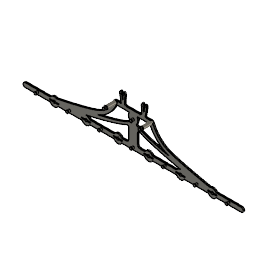
Piesa_4_cadru_sustinere (Autodesk Fusion 360 design; units mm, degrees)
part number: 2026-05-31-10-45-45-037
part number: 2026-05-31-14-30-49-266
Autodesk Fusion 360 part; units mm, degrees
sketch "top view" plane through (0, 0, 0) normal (0, 0, 1) x (1, 0, 0)
  line L0 (-248.6196, 9.3522) -> (-127.5156, 9.3522) construction
  line L1 (-248.6196, 9.3522) -> (-248.6196, 11.8522) construction
  arc A0 (-248.6196, 11.8522) -> (-249.2773, 6.9403) centre (-248.6196, 9.3522) ccw
  line L2 (-248.6196, 9.3522) -> (-216.3996, 9.3522) construction
  line L3 (-128.1733, 26.3643) -> (-128.1733, 29.0223) construction
  line L4 (-148.1733, 45.1233) -> (-148.1733, 43.1233) construction
  line L5 (-216.3996, 9.3522) -> (-216.3996, 13.6062) construction
  line L6 (-216.3996, 13.6062) -> (-213.7722, 13.6062) construction
  line L7 (-128.1733, 29.0223) -> (-180, 29.0223) construction
  spline S0 degree 5 poles (-213.7722, 13.6062) (-211.7009, 14.0329) (-207.6293, 14.8839) (-201.7349, 16.1535) (-194.3087, 17.832) (-185.8111, 19.9044) (-178.2122, 21.9474) (-171.6715, 23.9556) (-166.7674, 25.7797) (-163.881, 27.1788) (-162.3464, 28.1749) (-161.6154, 28.7858) (-161.3648, 29.0223) knots 0 0 0 0 0 0 0.1 0.2 0.3 0.4 0.5 0.6 0.7 0.76362 0.76362 0.76362 0.76362 0.76362 0.76362
  line L8 (-162.8508, 27.6198) -> (-159.8789, 30.4247)
  arc A1 (-170.1166, 24.5955) -> (-150.0471, 43.8225) centre (-180, 55) ccw
  line L9 (-132.8823, 41.1233) -> (-146.814, 41.1233)
  arc A2 (-148.1733, 45.1233) -> (-150.0471, 43.8225) centre (-148.1733, 43.1233) ccw
  line L10 (-128.1733, 41.1233) -> (-128.1733, 37.7953) construction
  line L11 (-128.1733, 35.7263) -> (-131.5853, 35.7263) construction
  line L12 (-128.1733, 41.1233) -> (-145.1293, 41.1233) construction
  line L13 (-145.1293, 41.1233) -> (-145.1293, 29.0223) construction
  line L14 (-180.8396, 9.3522) -> (-180.8396, 18.8752) construction
  line L15 (-180.8396, 18.8752) -> (-179.7346, 18.8752) construction
  arc A3 (-132.8823, 41.1233) -> (-131.5853, 32.7598) centre (-125.2153, 38.03) ccw
  arc A4 (-167.1807, 21.3913) -> (-165.0411, 22.2875) centre (-180, 55) ccw
  arc A5 (-158.8318, 25.9177) -> (-146.814, 41.1233) centre (-180, 55) ccw
  spline S1 degree 3 poles (-165.0411, 22.2875) (-163.9439, 22.76) (-162.9356, 23.2427) (-162.0149, 23.7457) (-160.8198, 24.3987) (-159.766, 25.0783) (-158.8318, 25.9177) knots 0.602738 0.602738 0.602738 0.602738 0.669843 0.669843 0.669843 0.756952 0.756952 0.756952 0.756952
  line L16 (-167.3845, 21.3116) -> (-167.4008, 21.3082)
  line L17 (-128.1733, 9.3522) -> (-128.1733, 26.3643) construction
  line L18 (-128.1733, 26.3643) -> (-134.6583, 26.3643) construction
  line L19 (-128.1733, 27.8213) -> (-135.0433, 27.8213) construction
  line L20 (-133.1518, 26.3643) -> (-133.1518, 2) construction
  arc A6 (-133.1518, 26.3643) -> (-135.0504, 27.8188) centre (-134.6583, 26.3643) ccw
  spline S2 degree 3 poles (-135.0504, 27.8188) (-135.0481, 27.8196) (-135.0457, 27.8204) (-135.0433, 27.8213) knots 0.499817 0.499817 0.499817 0.499817 0.499919 0.499919 0.499919 0.499919
  spline S3 degree 5 poles (-167.641, 21.24) (-166.401, 21.5014) (-163.424, 22.1424) (-158.8454, 23.181) (-152.9154, 24.6505) (-146.0504, 26.6065) (-140.0833, 28.6496) (-136.0679, 30.3417) (-133.5388, 31.6209) (-132.1186, 32.4368) (-131.5853, 32.7598) knots 0.130161 0.130161 0.130161 0.130161 0.130161 0.130161 0.2 0.3 0.4 0.5 0.6 0.664497 0.664497 0.664497 0.664497 0.664497 0.664497
  line L21 (-172.5766, 20.1992) -> (-162.7054, 22.2807)
  line L22 (-133.8581, 31.3829) -> (-129.3125, 34.1368)
  line L23 (-167.641, 21.24) -> (-167.1807, 21.3913)
  spline S4 degree 5 poles (-167.5607, 21.2747) (-167.5468, 21.2776) (-167.5328, 21.2805) (-167.5189, 21.2835) (-167.505, 21.2864) (-167.491, 21.2893) knots 0.123283 0.123283 0.123283 0.123283 0.123283 0.123283 0.124016 0.124016 0.124016 0.124016 0.124016 0.124016
  line L24 (-167.5678, 21.2732) -> (-167.5536, 21.2762)
  line L25 (-167.4981, 21.2878) -> (-167.4839, 21.2908)
  spline S5 degree 5 poles (-180.8396, 14.3522) (-179.0351, 14.7525) (-175.4777, 15.5549) (-170.2971, 16.764) (-163.7053, 18.3875) (-156.0341, 20.4372) (-149.0013, 22.5098) (-143.3292, 24.3981) (-139.4226, 25.8848) (-136.9109, 26.9566) (-135.5066, 27.6032) (-135.0504, 27.8188) knots 0 0 0 0 0 0 0.1 0.2 0.3 0.4 0.5 0.6 0.649903 0.649903 0.649903 0.649903 0.649903 0.649903
  line L26 (-138.104, 26.3752) -> (-131.9968, 29.2625)
  line L27 (-133.1518, 26.3643) -> (-133.1518, 14.3522)
  line L28 (-249.2773, 6.9403) -> (-220.7794, 6.9403)
  line L29 (-248.6196, 11.8522) -> (-220.7297, 11.8522)
  line L30 (-212.0198, 6.9403) -> (-185.2194, 6.9403)
  arc A7 (-185.2194, 6.9403) -> (-176.4598, 6.9403) centre (-180.8396, 9.3522) ccw
  arc A8 (-176.5095, 11.8522) -> (-180.8396, 14.3522) centre (-180.8396, 9.3522) ccw
  line L31 (-176.5095, 11.8522) -> (-149.6097, 11.8522)
  line L32 (-176.4598, 6.9403) -> (-149.6594, 6.9403)
  line L33 (-140.8998, 6.9403) -> (-128.1733, 6.9403)
  arc A9 (-149.6594, 6.9403) -> (-140.8998, 6.9403) centre (-145.2796, 9.3522) ccw
  arc A10 (-140.9495, 11.8522) -> (-149.6097, 11.8522) centre (-145.2796, 9.3522) ccw
  line L34 (-140.9495, 11.8522) -> (-135.6518, 11.8522)
  arc A11 (-135.6518, 11.8522) -> (-133.1518, 14.3522) centre (-135.6518, 14.3522) ccw
  arc A12 (-213.7722, 13.6062) -> (-220.7297, 11.8522) centre (-216.3996, 9.3522) ccw
  arc A13 (-220.7794, 6.9403) -> (-212.0198, 6.9403) centre (-216.3996, 9.3522) ccw
  line L35 (-128.1733, 45.1233) -> (-136.1553, 45.1233) construction
  line L36 (-148.1733, 45.1233) -> (-141.5903, 45.1233) construction
  line L37 (-136.1553, 45.1233) -> (-136.1553, 46.6233) construction
  line L38 (-140.4243, 45.1233) -> (-140.4243, 50.0803) construction
  line L39 (-140.4243, 50.0803) -> (-139.9633, 50.0803) construction
  line L40 (-140.4243, 50.0803) -> (-140.5759, 53.5518)
  line L41 (-140.4243, 50.0803) -> (-136.9203, 50.0803) construction
  line L42 (-139.5023, 50.0803) -> (-139.8213, 53.5851)
  line L43 (-139.5023, 50.0803) -> (-135.9583, 50.0803) construction
  line L44 (-140.2003, 53.5953) -> (-140.255, 54.8461) construction
  line L45 (-140.2003, 53.5953) -> (-138.9484, 53.5953) construction
  line L46 (-137.4093, 53.5851) -> (-137.6544, 46.6764)
  line L47 (-143.0856, 53.5518) -> (-141.5903, 45.1233)
  arc A14 (-140.4243, 50.0803) -> (-139.5099, 50.1635) centre (-139.9633, 50.0803) ccw
  arc A15 (-137.6544, 46.6764) -> (-136.1553, 45.1233) centre (-136.1553, 46.6233) ccw
  line L48 (-128.1733, 45.1233) -> (-136.1553, 45.1233)
  line L49 (-141.5903, 45.1233) -> (-148.1733, 45.1233)
  line L50 (-140.255, 54.8461) -> (-140.3137, 56.1783) construction
  line L51 (-140.3137, 56.1783) -> (-139.9454, 56.1428) construction
  line L52 (-140.3137, 56.1783) -> (-139.9437, 56.1783) construction
  line L53 (-139.9454, 56.1428) -> (-138.7329, 57.5625)
  line L54 (-139.9454, 56.1428) -> (-138.0784, 56.1428) construction
  line L55 (-140.3122, 56.1428) -> (-140.3124, 56.1428)
  line L56 (-140.6775, 56.1105) -> (-142.0103, 57.4179)
  arc A16 (-140.6777, 56.1108) -> (-140.5759, 53.5518) centre (-140.255, 54.8461) ccw
  arc A17 (-139.8213, 53.5851) -> (-139.9452, 56.1431) centre (-140.255, 54.8461) ccw
  arc A18 (-137.4093, 53.5851) -> (-138.7337, 57.5615) centre (-140.255, 54.8461) ccw
  arc A19 (-142.0094, 57.417) -> (-143.0856, 53.5518) centre (-140.255, 54.8461) ccw
  line L57 (-113.2611, 53.5518) -> (-114.7563, 45.1233)
  arc A20 (-113.2611, 53.5518) -> (-114.3373, 57.417) centre (-116.0917, 54.8461) ccw
  line L58 (-115.6692, 56.1105) -> (-114.3363, 57.4179)
  arc A21 (-115.7707, 53.5518) -> (-115.6689, 56.1108) centre (-116.0917, 54.8461) ccw
  arc A22 (-116.4014, 56.1431) -> (-116.5254, 53.5851) centre (-116.0917, 54.8461) ccw
  line L59 (-115.9223, 50.0803) -> (-115.7707, 53.5518)
  line L60 (-116.8443, 50.0803) -> (-116.5254, 53.5851)
  arc A23 (-116.8367, 50.1635) -> (-115.9223, 50.0803) centre (-116.3833, 50.0803) ccw
  arc A24 (-117.6129, 57.5615) -> (-118.9373, 53.5851) centre (-116.0917, 54.8461) ccw
  line L61 (-118.9373, 53.5851) -> (-118.6923, 46.6764)
  line L62 (-116.4012, 56.1428) -> (-117.6137, 57.5625)
  arc A25 (-120.1913, 45.1233) -> (-118.6923, 46.6764) centre (-120.1913, 46.6233) ccw
  line L63 (-128.1733, 45.1233) -> (-120.1913, 45.1233)
  line L64 (-114.7563, 45.1233) -> (-108.1733, 45.1233)
  arc A26 (-106.2995, 43.8225) -> (-108.1733, 45.1233) centre (-108.1733, 43.1233) ccw
  arc A27 (-106.2995, 43.8225) -> (-86.23, 24.5955) centre (-76.3466, 55) ccw
  spline S6 degree 5 poles (-42.5745, 13.6062) (-44.6458, 14.0329) (-48.7173, 14.8839) (-54.6117, 16.1535) (-62.0379, 17.832) (-70.5356, 19.9044) (-78.1344, 21.9474) (-84.6752, 23.9556) (-89.5793, 25.7797) (-92.4656, 27.1788) (-94.0003, 28.1749) (-94.7313, 28.7858) (-94.9818, 29.0223) knots 0 0 0 0 0 0 0.1 0.2 0.3 0.4 0.5 0.6 0.7 0.76362 0.76362 0.76362 0.76362 0.76362 0.76362
  line L65 (-221.9985, 11.9116) -> (-205.5458, 15.3008)
  line L66 (-34.3481, 11.9116) -> (-50.8008, 15.3008)
  line L67 (-93.4959, 27.6198) -> (-96.4677, 30.4247)
  arc A28 (-35.6169, 11.8522) -> (-42.5745, 13.6062) centre (-39.947, 9.3522) ccw
  line L68 (-7.727, 11.8522) -> (-35.6169, 11.8522)
  arc A29 (-7.0693, 6.9403) -> (-7.727, 11.8522) centre (-7.727, 9.3522) ccw
  line L69 (-7.0693, 6.9403) -> (-35.5672, 6.9403)
  arc A30 (-44.3268, 6.9403) -> (-35.5672, 6.9403) centre (-39.947, 9.3522) ccw
  line L70 (-44.3268, 6.9403) -> (-71.1272, 6.9403)
  arc A31 (-79.8868, 6.9403) -> (-71.1272, 6.9403) centre (-75.507, 9.3522) ccw
  arc A32 (-75.507, 14.3522) -> (-79.8372, 11.8522) centre (-75.507, 9.3522) ccw
  spline S7 degree 5 poles (-75.507, 14.3522) (-77.3116, 14.7525) (-80.8689, 15.5549) (-86.0495, 16.764) (-92.6413, 18.3875) (-100.3125, 20.4372) (-107.3453, 22.5098) (-113.0174, 24.3981) (-116.9241, 25.8848) (-119.4357, 26.9566) (-120.8401, 27.6032) (-121.2962, 27.8188) knots 0 0 0 0 0 0 0.1 0.2 0.3 0.4 0.5 0.6 0.649903 0.649903 0.649903 0.649903 0.649903 0.649903
  line L71 (-186.8976, 13.0084) -> (-174.7816, 15.6959)
  line L72 (-69.4491, 13.0084) -> (-81.565, 15.6959)
  line L73 (-118.2426, 26.3752) -> (-124.3498, 29.2625)
  line L74 (-79.8372, 11.8522) -> (-106.7369, 11.8522)
  line L75 (-79.8868, 6.9403) -> (-106.6872, 6.9403)
  arc A33 (-115.4468, 6.9403) -> (-106.6872, 6.9403) centre (-111.067, 9.3522) ccw
  arc A34 (-106.7369, 11.8522) -> (-115.3972, 11.8522) centre (-111.067, 9.3522) ccw
  line L76 (-115.3972, 11.8522) -> (-120.6948, 11.8522)
  arc A35 (-123.1948, 14.3522) -> (-120.6948, 11.8522) centre (-120.6948, 14.3522) ccw
  line L77 (-123.1948, 26.3643) -> (-123.1948, 14.3522)
  arc A36 (-121.2962, 27.8188) -> (-123.1948, 26.3643) centre (-121.6883, 26.3643) ccw
  line L78 (-115.4468, 6.9403) -> (-128.1733, 6.9403)
  spline S8 degree 5 poles (-88.7056, 21.24) (-89.9456, 21.5014) (-92.9226, 22.1424) (-97.5012, 23.181) (-103.4313, 24.6505) (-110.2963, 26.6065) (-116.2634, 28.6496) (-120.2787, 30.3417) (-122.8079, 31.6209) (-124.2281, 32.4368) (-124.7613, 32.7598) knots 0.130161 0.130161 0.130161 0.130161 0.130161 0.130161 0.2 0.3 0.4 0.5 0.6 0.664497 0.664497 0.664497 0.664497 0.664497 0.664497
  line L79 (-83.77, 20.1992) -> (-93.6413, 22.2807)
  line L80 (-122.4885, 31.3829) -> (-127.0341, 34.1368)
  arc A37 (-109.5327, 41.1233) -> (-97.5149, 25.9177) centre (-76.3466, 55) ccw
  spline S9 degree 3 poles (-91.3055, 22.2875) (-92.4027, 22.76) (-93.4111, 23.2427) (-94.3317, 23.7457) (-95.5268, 24.3987) (-96.5806, 25.0783) (-97.5149, 25.9177) knots 0.602738 0.602738 0.602738 0.602738 0.669843 0.669843 0.669843 0.756952 0.756952 0.756952 0.756952
  arc A38 (-91.3055, 22.2875) -> (-89.1659, 21.3913) centre (-76.3466, 55) ccw
  line L81 (-88.7056, 21.24) -> (-89.1659, 21.3913)
  line L82 (-123.4643, 41.1233) -> (-109.5327, 41.1233)
  arc A39 (-124.7613, 32.7598) -> (-123.4643, 41.1233) centre (-131.1313, 38.03) ccw
  line L83 (-128.1733, 41.1233) -> (-128.1733, 130) construction
  line L84 (-128.1733, 41.1233) -> (-128.1733, 130) construction
  line L85 (-128.1733, 27.8213) -> (-128.1733, 29.0223) construction
  circle A40 centre (-148.1733, 43.1233) radius 1.5
  circle A41 centre (-108.1733, 43.1233) radius 1.5
  line L86 (-131.5853, 32.7598) -> (-128.4593, 32.7598) construction
  line L87 (-128.1733, 45.1233) -> (-128.1733, 36.2953) construction
  circle A42 centre (-128.1733, 36.2953) radius 1.5
  circle A43 centre (-128.1733, 9.4403) radius 1.5
  line L88 (-128.1733, 6.9403) -> (-128.1733, 10.9403) construction
  circle A44 centre (-92.6133, 9.4403) radius 1.5
  circle A45 centre (-57.0533, 9.4403) radius 1.5
  circle A46 centre (-21.4933, 9.4403) radius 1.5
  circle A47 centre (-163.7333, 9.4403) radius 1.5
  circle A48 centre (-199.2933, 9.4403) radius 1.5
  circle A49 centre (-234.8533, 9.4403) radius 1.5
  circle A50 centre (-148.1733, 43.1233) radius 1.25
  circle A51 centre (-108.1733, 43.1233) radius 1.25
  circle A52 centre (-128.1733, 36.2953) radius 1.25
  circle A53 centre (-128.1733, 9.4403) radius 1.25
  circle A54 centre (-163.7333, 9.4403) radius 1.25
  circle A55 centre (-199.2933, 9.4403) radius 1.25
  circle A56 centre (-234.8533, 9.4403) radius 1.25
  circle A57 centre (-92.6133, 9.4403) radius 1.25
  circle A58 centre (-57.0533, 9.4403) radius 1.25
  circle A59 centre (-21.4933, 9.4403) radius 1.25
  line L89 (-180.8396, 9.3522) -> (-185.6136, 9.3522) construction
  line L90 (-185.6136, 9.3522) -> (-185.6136, 9.8132) construction
  line L91 (-185.6136, 9.8132) -> (-182.2202, 9.8132)
  line L92 (-185.6136, 8.8912) -> (-182.2202, 8.8912)
  arc A60 (-185.6136, 9.8132) -> (-185.6136, 8.8912) centre (-185.6136, 9.3522) ccw
  line L93 (-176.0656, 9.8132) -> (-179.459, 9.8132)
  line L94 (-176.0656, 8.8912) -> (-179.459, 8.8912)
  arc A61 (-176.0656, 8.8912) -> (-176.0656, 9.8132) centre (-176.0656, 9.3522) ccw
  arc A62 (-182.2202, 8.8912) -> (-179.459, 8.8912) centre (-180.8396, 9.3522) ccw
  arc A63 (-179.459, 9.8132) -> (-182.2202, 9.8132) centre (-180.8396, 9.3522) ccw
  line L95 (-180.8396, 9.3522) -> (-145.2796, 9.3522) construction
  line L96 (-163.0596, 9.3522) -> (-163.0596, 17) construction
  line L97 (-150.0536, 8.8912) -> (-146.6602, 8.8912)
  line L98 (-150.0536, 9.8132) -> (-146.6602, 9.8132)
  line L99 (-140.5056, 8.8912) -> (-143.899, 8.8912)
  line L100 (-140.5056, 9.8132) -> (-143.899, 9.8132)
  arc A64 (-150.0536, 9.8132) -> (-150.0536, 8.8912) centre (-150.0536, 9.3522) ccw
  arc A65 (-140.5056, 8.8912) -> (-140.5056, 9.8132) centre (-140.5056, 9.3522) ccw
  arc A66 (-146.6602, 8.8912) -> (-143.899, 8.8912) centre (-145.2796, 9.3522) ccw
  arc A67 (-143.899, 9.8132) -> (-146.6602, 9.8132) centre (-145.2796, 9.3522) ccw
  line L101 (-216.3996, 9.3522) -> (-180.8396, 9.3522) construction
  line L102 (-198.6196, 9.3522) -> (-198.6196, 14.7055) construction
  line L103 (-221.1736, 9.8132) -> (-217.7802, 9.8132)
  arc A68 (-221.1736, 9.8132) -> (-221.1736, 8.8912) centre (-221.1736, 9.3522) ccw
  line L104 (-221.1736, 8.8912) -> (-217.7802, 8.8912)
  line L105 (-211.6256, 9.8132) -> (-215.019, 9.8132)
  arc A69 (-211.6256, 8.8912) -> (-211.6256, 9.8132) centre (-211.6256, 9.3522) ccw
  line L106 (-211.6256, 8.8912) -> (-215.019, 8.8912)
  arc A70 (-215.019, 9.8132) -> (-217.7802, 9.8132) centre (-216.3996, 9.3522) ccw
  arc A71 (-217.7802, 8.8912) -> (-215.019, 8.8912) centre (-216.3996, 9.3522) ccw
  line L107 (-115.841, 8.8912) -> (-112.4476, 8.8912)
  arc A72 (-115.841, 9.8132) -> (-115.841, 8.8912) centre (-115.841, 9.3522) ccw
  line L108 (-115.841, 9.8132) -> (-112.4476, 9.8132)
  line L109 (-106.293, 8.8912) -> (-109.6865, 8.8912)
  arc A73 (-106.293, 8.8912) -> (-106.293, 9.8132) centre (-106.293, 9.3522) ccw
  line L110 (-106.293, 9.8132) -> (-109.6865, 9.8132)
  line L111 (-80.281, 9.8132) -> (-76.8876, 9.8132)
  arc A74 (-80.281, 9.8132) -> (-80.281, 8.8912) centre (-80.281, 9.3522) ccw
  line L112 (-80.281, 8.8912) -> (-76.8876, 8.8912)
  line L113 (-70.733, 9.8132) -> (-74.1265, 9.8132)
  arc A75 (-70.733, 8.8912) -> (-70.733, 9.8132) centre (-70.733, 9.3522) ccw
  line L114 (-70.733, 8.8912) -> (-74.1265, 8.8912)
  line L115 (-44.721, 9.8132) -> (-41.3276, 9.8132)
  arc A76 (-44.721, 9.8132) -> (-44.721, 8.8912) centre (-44.721, 9.3522) ccw
  line L116 (-44.721, 8.8912) -> (-41.3276, 8.8912)
  line L117 (-35.173, 9.8132) -> (-38.5665, 9.8132)
  arc A77 (-35.173, 8.8912) -> (-35.173, 9.8132) centre (-35.173, 9.3522) ccw
  line L118 (-35.173, 8.8912) -> (-38.5665, 8.8912)
  arc A78 (-109.6865, 9.8132) -> (-112.4476, 9.8132) centre (-111.067, 9.3522) ccw
  arc A79 (-112.4476, 8.8912) -> (-109.6865, 8.8912) centre (-111.067, 9.3522) ccw
  arc A80 (-74.1265, 9.8132) -> (-76.8876, 9.8132) centre (-75.507, 9.3522) ccw
  arc A81 (-76.8876, 8.8912) -> (-74.1265, 8.8912) centre (-75.507, 9.3522) ccw
  arc A82 (-38.5665, 9.8132) -> (-41.3276, 9.8132) centre (-39.947, 9.3522) ccw
  arc A83 (-41.3276, 8.8912) -> (-38.5665, 8.8912) centre (-39.947, 9.3522) ccw
  circle A84 centre (-148.1733, 43.1233) radius 2
  circle A85 centre (-108.1733, 43.1233) radius 2
  point P0 (-161.3648, 29.0223)
  point P1 (-150.0536, 9.3522)
  point P2 (-140.5056, 9.3522)
  dimension "d1" = 121.104
  dimension "d2" = 2.5
  dimension "d3" = 5
  dimension "d5" = 121.104
  dimension "d6" = 32.22
  dimension "d7" = 2.911
  dimension "d8" = 10
  dimension "d13" = 38.183
  dimension "d14" = 20
  dimension "d15" = 2
  dimension "d16" = 4
  dimension "d17" = 4.254
  dimension "d18" = 63.941
  dimension "d19" = 16.101
  dimension "d22" = 4
  dimension "d23" = 4.709
  dimension "d25" = 5.397
  dimension "d26" = 3.412
  dimension "d28" = 16.956
  dimension "d29" = 12.101
  dimension "d30" = 9.523
  dimension "d31" = 1.105
  dimension "d35" = 16.535
  dimension "d36" = 19.424
  dimension "d37" = 6.485
  dimension "d38" = 3.013
  dimension "d39" = 1.457
  dimension "d40" = 6.87
  dimension "d41" = 5
  dimension "d42" = 7.982
  dimension "d43" = 6.583
  dimension "d44" = 1.5
  dimension "d45" = 3
  dimension "d46" = 1.166
  dimension "d47" = 4.957
  dimension "d49" = 0.461
  dimension "d50" = 0.922
  dimension "d51" = 92.5
  dimension "d53" = 95.2
  dimension "d55" = 92.5
  dimension "d56" = 1.252
  dimension "d57" = 2.667
  dimension "d58" = 6.225
  dimension "d59" = 0.37
  dimension "d60" = 5.5
  dimension "d61" = 49.5
  dimension "d62" = 1.867
  dimension "d63" = 0.367
  dimension "d64" = 3
  dimension "d65" = 3
  dimension "d66" = 3.126
  dimension "d67" = 8.828
  dimension "d68" = 3
  dimension "d69" = 26.855
  dimension "d70" = 3
  dimension "d73" = 106.68
  dimension "d74" = 0
  dimension "d77" = -106.68
  dimension "d78" = 0
  dimension "d79" = 2.5
  dimension "d80" = 2.5
  dimension "d81" = 2.5
  dimension "d82" = 2.5
  dimension "d83" = 2.5
  dimension "d84" = 2.5
  dimension "d85" = 2.5
  dimension "d86" = 2.5
  dimension "d87" = 2.5
  dimension "d88" = 2.5
  dimension "d89" = 4.774
  dimension "d90" = 0.461
  dimension "d91" = 0.922
  dimension "d94" = 4
  dimension "d95" = 4
  constraint horizontal L0
  constraint perpendicular L0 L1
  constraint coincident L0.start L1.start
  constraint perpendicular L1 L29
  constraint parallel L0 L28
  constraint coincident L2.end L5.start
  constraint concentric A12 A70
  constraint perpendicular L0 L3
  constraint perpendicular L48 L83
  constraint perpendicular L4 L49
  constraint coincident L4.end A2.centre
  constraint perpendicular L2 L5
  constraint perpendicular L5 L6
  constraint tangent A1 A2
  constraint coincident P0 A1
  constraint coincident L7 P0
  constraint coincident P0 S0.end
  constraint midpoint P0 L8
  constraint coincident S0 A1.start
  constraint concentric A1 A4
  constraint perpendicular L9 L10
  constraint perpendicular L3 L11
  constraint perpendicular L7 L13
  constraint coincident L14.start A7.centre
  constraint perpendicular L14 L31
  constraint perpendicular L14 L15
  constraint concentric A4 A5
  constraint perpendicular L17 L33
  constraint perpendicular L17 L18
  constraint coincident L18.end A6.centre
  constraint perpendicular L19 L85
  constraint coincident L18 L20.start
  constraint tangent L20 A6
  constraint coincident A6 S2.start
  constraint midpoint S3.start L21
  constraint midpoint A3.end L22
  constraint coincident L23 S4.end
  constraint midpoint S4.start L24
  constraint midpoint S4.end L25
  constraint coincident L14 S5.start
  constraint midpoint A6.end L26
  constraint collinear L28 L30
  constraint collinear L29 L31
  constraint collinear L30 L32
  constraint concentric A7 A8
  constraint collinear L31 L34
  constraint collinear L32 L33
  constraint concentric A9 A10
  constraint tangent L20 A11
  constraint tangent L34 A11
  constraint concentric A12 A13
  constraint perpendicular L35 L83
  constraint perpendicular L4 L36
  constraint perpendicular L35 L37
  constraint coincident L37.end A15.centre
  constraint perpendicular L38 L49
  constraint perpendicular L38 L39
  constraint coincident L39.end A14.centre
  constraint horizontal L41
  constraint horizontal L43
  constraint coincident L42.start A14
  constraint coincident L41 L42.start
  constraint horizontal L45
  constraint coincident L44.end L50.start
  constraint concentric A17 A18
  constraint tangent L46 A15
  constraint coincident L42 A14.end
  constraint collinear L48 L49
  constraint horizontal L52
  constraint horizontal L54
  constraint horizontal L55
  constraint coincident L50 L55.start
  constraint symmetric L50 L51.end L56.start
  constraint symmetric L50 L53.end L56.end
  constraint coincident L56 A16.start
  constraint coincident L53 A17.end
  constraint coincident L53 A18.end
  constraint coincident L56 A19.start
  constraint concentric A18 A19
  constraint midpoint L6.end L65
  constraint midpoint S5.start L71
  constraint symmetric L35.start L48.start L83
  constraint symmetric L4.start L64.end L83
  constraint symmetric P0 S6.end L85
  constraint symmetric L8.start L67.start L85
  constraint symmetric L8.end L67.end L85
  constraint symmetric A1.end A26.start L83
  constraint symmetric A1 A27 L83
  constraint symmetric L9.end A37.start L83
  constraint symmetric A2 A26 L83
  constraint symmetric L9.start L82.start L83
  constraint symmetric A3.end S8.end L85
  constraint symmetric A3 A39 L85
  constraint symmetric A5 A37 L83
  constraint symmetric A6.end S7.end L85
  constraint symmetric L22.start L80.start L85
  constraint symmetric L22.end L80.end L85
  constraint symmetric L26.end L73.end L85
  constraint symmetric L35.end A25.start L83
  constraint symmetric L36.end L57.end L83
  constraint symmetric L38.end L59.start L83
  constraint symmetric L42.start L60.start L83
  constraint symmetric L42.end A22.end L83
  constraint symmetric L40.end A21.start L83
  constraint symmetric L46.start A24.end L83
  constraint symmetric L46.end L61.end L83
  constraint symmetric L47.start L57.start L83
  constraint symmetric A14.end A23.start L83
  constraint symmetric A14 A23 L83
  constraint symmetric A15 A25 L83
  constraint symmetric L51.end L62.start L83
  constraint symmetric L53.end L62.end L83
  constraint symmetric L56.start L58.start L83
  constraint symmetric L56.end L58.end L83
  constraint symmetric A16.start A21.end L83
  constraint symmetric A16 A21 L83
  constraint symmetric A17.end A22.start L83
  constraint symmetric A17 A22 L83
  constraint symmetric A18.end A24.start L83
  constraint symmetric A19.start A20.end L83
  constraint symmetric A18 A24 L83
  constraint symmetric A19 A20 L83
  constraint collinear L83 L85
  constraint coincident L0 L17.start
  constraint concentric A26 A41
  constraint perpendicular L33 L87
  constraint coincident L87.end A42.centre
  constraint coincident A43 L88.end
  constraint coincident A42 L10.end
  constraint concentric A40 A50
  constraint concentric A41 A51
  constraint concentric A42 A52
  constraint concentric A43 A53
  constraint concentric A47 A54
  constraint concentric A48 A55
  constraint concentric A49 A56
  constraint concentric A44 A57
  constraint concentric A45 A58
  constraint concentric A46 A59
  constraint perpendicular L14 L89
  constraint perpendicular L89 L90
  constraint coincident L89.end L90.start
  constraint perpendicular L14 L91
  constraint tangent L92 A60
  constraint parallel L0 L92
  constraint symmetric L14 L90.end L93.start
  constraint symmetric L14 L92.start L94.start
  constraint symmetric L14 A60 A61
  constraint symmetric L14 L91.end L93.end
  constraint symmetric L14 L92.end L94.end
  constraint concentric A62 A63
  constraint coincident A9.centre A10.centre
  constraint parallel L0 L95
  constraint midpoint L95 L96.start
  constraint perpendicular L31 L96
  constraint symmetric L90.end L96 L100.start
  constraint symmetric L89.end L96 P2
  constraint symmetric L92.start L96 L99.start
  constraint symmetric L91.end L96 L100.end
  constraint symmetric L92.end L96 L99.end
  constraint symmetric L93.start L96 L98.start
  constraint symmetric L93.end L96 L98.end
  constraint symmetric L94.start L96 L97.start
  constraint symmetric L94.end L96 L97.end
  constraint symmetric A61.centre L96 P1
  constraint symmetric A60 L96 A65
  constraint symmetric A61 L96 A64
  constraint concentric A66 A67
  constraint perpendicular L14 L101
  constraint midpoint L101 L102.start
  constraint perpendicular L101 L102
  constraint symmetric L90.end L102 L105.start
  constraint symmetric L92.start L102 A69.start
  constraint symmetric A60 L102 A69
  constraint symmetric L91.end L102 L105.end
  constraint symmetric L92.end L102 L106.end
  constraint symmetric L93.start L102 L103.start
  constraint symmetric L93.end L102 L103.end
  constraint symmetric L94.start L102 A68.end
  constraint symmetric L94.end L102 L104.end
  constraint symmetric A61 L102 A68
  constraint concentric A70 A71
  constraint symmetric L17 L90.end L113.start
  constraint symmetric L17 L92.start A75.start
  constraint symmetric L17 A60 A75
  constraint symmetric L17 L91.end L113.end
  constraint symmetric L17 L92.end L114.end
  constraint symmetric L17 L93.start L111.start
  constraint symmetric L17 L93.end L111.end
  constraint symmetric L17 L94.start A74.end
  constraint symmetric L17 L94.end L112.end
  constraint symmetric L17 A61 A74
  constraint symmetric L17 L97.start L109.start
  constraint symmetric L17 L97.end L109.end
  constraint symmetric L17 L98.start A73.end
  constraint symmetric L17 L98.end L110.end
  constraint symmetric L17 L99.start L107.start
  constraint symmetric L17 L99.end L107.end
  constraint symmetric L17 L100.start A72.start
  constraint symmetric L17 L100.end L108.end
  constraint symmetric L17 A64 A73
  constraint symmetric L17 A65 A72
  constraint symmetric L17 L103.start L117.start
  constraint symmetric L17 L103.end L117.end
  constraint symmetric L17 A68.end A77.start
  constraint symmetric L17 A68 A77
  constraint symmetric L17 L104.end L118.end
  constraint symmetric L17 L105.start L115.start
  constraint symmetric L17 L105.end L115.end
  constraint symmetric L17 A69.start A76.end
  constraint symmetric L17 A69 A76
  constraint symmetric L17 L106.end L116.end
  constraint concentric A78 A79
  constraint concentric A80 A81
  constraint concentric A82 A83
  constraint concentric A50 A84
  constraint concentric A41 A85
  measures "d1" distance of L0.start L0.end
  measures "d2" distance of L0.start L1.end
  measures "d3" diameter of A0
  measures "d5" distance of A0.end L33.end
  measures "d6" distance of L0.start L2.end
  measures "d7" diameter of A70
  measures "d8" diameter of A12
  measures "d13" distance of L33.end L35.start
  measures "d14" distance of L35.start L4.start
  measures "d15" distance of L4.start L4.end
  measures "d16" diameter of A2
  measures "d17" distance of L2.end L5.end
  measures "d18" diameter of A1
  measures "d19" distance of L35.start L3.end
  measures "d22" distance of L35.start L10.start
  measures "d23" distance of L10.start L9.start
  measures "d25" distance of L10.start L11.start
  measures "d26" distance of L11.start L11.end
  measures "d28" distance of L10.start L12.end
  measures "d29" distance of L12.end L13.end
  measures "d30" distance of L14.start L14.end
  measures "d31" distance of L14.end L15.end
  measures "d35" diameter of A3
  measures "d36" distance of L33.end L3.start
  measures "d37" distance of L3.start L18.end
  measures "d38" diameter of A6
  measures "d39" distance of L3.start L19.start
  measures "d40" distance of L19.start L19.end
  measures "d41" diameter of A11
  measures "d42" distance of L35.start L35.end
  measures "d43" distance of L4.start L36.end
  measures "d44" distance of L35.end L37.end
  measures "d45" diameter of A15
  measures "d46" distance of L36.end L38.start
  measures "d47" distance of L38.start L38.end
  measures "d49" distance of L38.end L39.end
  measures "d50" diameter of A14
  measures "d51" angle of L40 L41
  measures "d53" angle of L42 L43
  measures "d55" angle of L44 L45
  measures "d56" distance of L44.start L44.end
  measures "d57" diameter of A17
  measures "d58" diameter of A18
  measures "d59" distance of L50.end L51.end
  measures "d60" angle of L51 L52
  measures "d61" angle of L53 L54
  measures "d62" distance of L51.end L53.end
  measures "d63" distance of L51.end L55.end
  measures "d64" diameter of A40
  measures "d65" diameter of A41
  measures "d66" distance of A3.end L86.end
  measures "d67" distance of L35.start L87.end
  measures "d68" diameter of A42
  measures "d69" distance of L87.end A43.centre
  measures "d70" diameter of A43
  measures "d79" diameter of A50
  measures "d80" diameter of A51
  measures "d81" diameter of A52
  measures "d82" diameter of A53
  measures "d83" diameter of A54
  measures "d84" diameter of A55
  measures "d85" diameter of A56
  measures "d86" diameter of A57
  measures "d87" diameter of A58
  measures "d88" diameter of A59
  measures "d89" distance of L14.start L89.end
  measures "d90" distance of L89.end L90.end
  measures "d91" diameter of A60
  measures "d94" diameter of A84
  measures "d95" diameter of A85
extrude "Extrude1" add sketch "top view" along normal blind 1.5 contours A0 S0 A1 L28 L29 L30 A7 L32 L33 A9 A12 A13 L40 L42 L46 L47 A14 A15 L48 L49 L53 L56 A16 A17 A18 A19 L57 A20 L58 A21 A22 L59 L60 A23 A24 L61 L62 A25 L63 L64 A27 S6 L65 L66 A28 L68 A29 L69 A30 L70 A31 L75 A33 L78 A84 A85 | A12 L65 | A2 A84 | L66 A28 | A26 A85 makes body 1
extrude "Extrude2" add sketch "top view" along normal blind 12 contours A2 A84 | A26 A85 | A40 | A41 | A50 | A51 bodies 1
extrude "Extrude3" add sketch "top view" along normal blind 1.75 from surface at 12 contours A50 | A51 bodies 1
sketch "sectiune suporti" plane through (0, 0, 0) normal (0, 0, 1) x (1, 0, 0)
  line L0 (16, 11) -> (16, 10.24)
  line L1 (16, 10.24) -> (17.25, 10.24)
  line L2 (16, 11) -> (17.5, 11)
  arc A0 (17.25, 10.24) -> (17.5, 11) centre (15.7079, 11.1684) ccw
  dimension "d102" = 0.76
  dimension "d103" = 1.25
  dimension "d104" = 1.5
  dimension "d106" = 3.6
  constraint vertical L0
  constraint perpendicular L0 L1
  constraint perpendicular L0 L2
  measures "d102" distance of L0.start L0.end
  measures "d103" distance of L0.end L1.end
  measures "d104" distance of L0.start L2.end
  measures "d106" diameter of A0
revolve "Revolve1" add sketch "sectiune suporti" angle 360 about axis through (16, 11, 0) along (0, -1, 0) separate body makes body 2
move_body "Move1" bodies 2 to x (1, 0, 0) y (0, 0, 1) z (0, -1, 0) at (0, 10.24, -10.24)
copy_body "CopyPasteBodies1" bodies 2 makes body 3
move_body "Move2" bodies 3 to x (1, 0, 0) y (0, 1, 0) z (0, 0, 1) at (-164.1733, 32.8833, 13.75)
move_body "Move3" bodies 2 to x (1, 0, 0) y (0, 1, 0) z (0, 0, 1) at (0, 0, 9)
copy_body "CopyPasteBodies2" bodies 2 makes body 4
move_body "Move4" bodies 4 to x (1, 0, 0) y (0, 1, 0) z (0, 0, 1) at (-124.1733, 32.8833, 4.75)
extrude "Extrude4" add sketch "top view" along normal blind 1.5 contours A42 | A43 | A44 | A45 | A46 | A47 | A48 | A49 | A52 | A53 | A54 | A55 | A56 | A57 | A58 | A59 bodies 1
extrude "Extrude5" add sketch "top view" along normal blind 2 from surface at 1.5 contours A52 | A53 | A54 | A55 | A56 | A57 | A58 | A59 bodies 1
copy_body "CopyPasteBodies3" bodies 2 makes body 5
move_body "Move5" bodies 5 to x (1, 0, 0) y (0, 1, 0) z (0, 0, 1) at (-37.4933, -0.7997, -5.5)
copy_body "CopyPasteBodies4" bodies 2 makes body 6
move_body "Move6" bodies 6 to x (1, 0, 0) y (0, 1, 0) z (0, 0, 1) at (-73.0533, -0.7997, -5.5)
copy_body "CopyPasteBodies5" bodies 2 makes body 7
move_body "Move7" bodies 7 to x (1, 0, 0) y (0, 1, 0) z (0, 0, 1) at (-108.6133, -0.7997, -5.5)
copy_body "CopyPasteBodies6" bodies 2 makes body 8
move_body "Move8" bodies 8 to x (1, 0, 0) y (0, 1, 0) z (0, 0, 1) at (-144.1733, -0.7997, -5.5)
copy_body "CopyPasteBodies7" bodies 2 makes body 9
move_body "Move9" bodies 9 to x (1, 0, 0) y (0, 1, 0) z (0, 0, 1) at (-144.1733, 26.0553, -5.5)
copy_body "CopyPasteBodies8" bodies 2 makes body 10
move_body "Move10" bodies 10 to x (1, 0, 0) y (0, 1, 0) z (0, 0, 1) at (-179.7333, -0.7997, -5.5)
copy_body "CopyPasteBodies9" bodies 2 makes body 11
move_body "Move11" bodies 11 to x (1, 0, 0) y (0, 1, 0) z (0, 0, 1) at (-215.2933, -0.7997, -5.5)
move_body "Move12" bodies 2 to x (1, 0, 0) y (0, 1, 0) z (0, 0, 1) at (-250.8533, -0.7997, -5.5)
copy_body "Body->Comp1" bodies 1 removing the originals makes body 12 in component "Piesa_4 (1)"
copy_body "CutPasteBodies1" bodies 2 removing the originals makes body 13 in component "Piesa_4 (1)"
copy_body "CutPasteBodies2" bodies 3 removing the originals makes body 14 in component "Piesa_4 (1)"
copy_body "CutPasteBodies3" bodies 4 removing the originals makes body 15 in component "Piesa_4 (1)"
copy_body "CutPasteBodies4" bodies 5 removing the originals makes body 16 in component "Piesa_4 (1)"
copy_body "CutPasteBodies5" bodies 6 removing the originals makes body 17 in component "Piesa_4 (1)"
copy_body "CutPasteBodies6" bodies 7 removing the originals makes body 18 in component "Piesa_4 (1)"
copy_body "CutPasteBodies7" bodies 8 removing the originals makes body 19 in component "Piesa_4 (1)"
copy_body "CutPasteBodies8" bodies 9 removing the originals makes body 20 in component "Piesa_4 (1)"
copy_body "CutPasteBodies9" bodies 10 removing the originals makes body 21 in component "Piesa_4 (1)"
copy_body "CutPasteBodies10" bodies 11 removing the originals makes body 22 in component "Piesa_4 (1)"
component "Piesa_4 (1)" placed x (1, 0, 0) y (0, 1, 0) z (0, 0, 1) at (0, 0, 0)
equation "d47 = 4.936 mm + 0.021 mm"
equation "d50 = 0.461 mm + 0.461 mm"
equation "d73 = 35.56 mm + 35.56 mm + 35.56 mm"
equation "d77 = -35.56 mm - 35.56 mm - 35.56 mm"
equation "d91 = 0.461 mm + 0.461 mm"
named bodies: "cadru principal", "capat suport", "capat suport 1", "capat suport 2", "capat suport 3", "capat suport 4", "capat suport 5", "capat suport 6", "capat suport 7", "capat suport 8", "capat suport 9"
